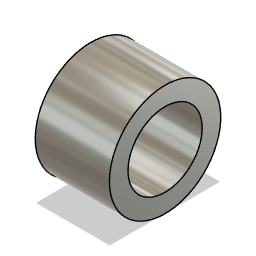
12x20x12 bushing v4 (Autodesk Fusion 360 design; units mm, degrees)
Autodesk Fusion 360 part; units mm, degrees
sketch "Sketch1" plane through (0, 0, 0) normal (1, 0, 0) x (0, 0, -1)
  circle A0 centre (0, 0) radius 6
  circle A1 centre (0, 0) radius 9
  dimension "d1" = 12
  dimension "d2" = 18
  constraint coincident A0.centre A1.centre
  constraint concentric A0 A1
  measures "d1" diameter of A0
  measures "d2" diameter of A1
extrude "Extrude1" add sketch "Sketch1" along normal blind 12 makes body 1
copy_body "Body->Comp1" bodies 1 removing the originals makes body 2 in component "12x18x12 bushing"
component "12x18x12 bushing" placed x (1, 0, 0) y (0, 1, 0) z (0, 0, 1) at (0, 0, 0)
named bodies: "12x22x22 bushing", "12x18x12 bushing"
